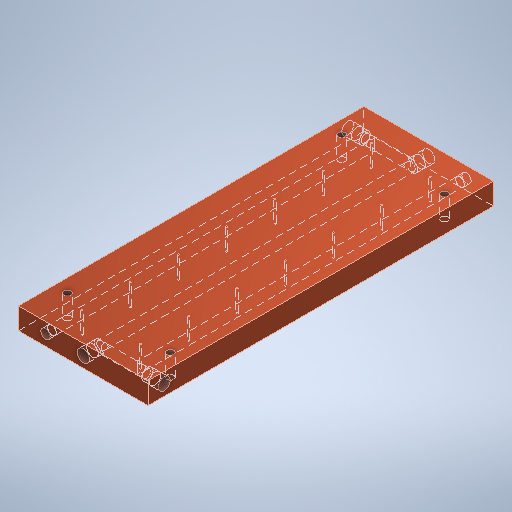
# Autodesk Inventor part: Cold Plate
Saved by Autodesk Inventor 2025 (Build 290162000, 162)
## iProperties
Created: 2025-06-10
Part Number: Cold Plate
Material: Copper
Document SubType Name: Modeling
Designer: Caleb Fangmeier
Density: 8.94 g/cm^3
Appearance: Copper - Satin
Author: Caleb Fangmeier
Autodesk Inventor part; units mm, degrees
ref_plane "YZ Plane" through (0, 0, 0) normal (1, 0, 0) x (0, 1, 0)
ref_plane "XZ Plane" through (0, 0, 0) normal (0, 1, 0) x (-1, 0, 0)
ref_plane "XY Plane" through (0, 0, 0) normal (0, 0, 1) x (1, 0, 0)
sketch "Sketch1" plane through (0, 0, 0) normal (0, 1, 0) x (-1, 0, 0)
  line L0 (-60, -160) -> (60, -160)
  line L1 (60, -160) -> (60, 160)
  line L2 (60, 160) -> (-60, 160)
  line L3 (-60, 160) -> (-60, -160)
  line L4 (-60, -160) -> (60, 160) construction
  line L5 (60, -160) -> (-60, 160) construction
  point P0 (0, 0)
  dimension "d0" = 120
  dimension "d1" = 320
  constraints: 12 end point, 2 midpoint, 2 parallel, 1 horizontal, 1 perpendicular
  measures "d0" distance of L2.end L1.end
  measures "d1" distance of L0.end L1.end
extrude "Extrusion1" add sketch "Sketch1" along normal blind 20
sketch "Right Center Hole and Plug" plane through (-60, 0, 160) normal (0, 0, 1) x (1, 0, 0)
  line L0 (120, 0) -> (120, 20) projected
  line L1 (0, 0) -> (120, 0) projected
  point P0 (60, 0)
  point P1 (60, 10)
  dimension "d4" = 60
  dimension "d5" = 10
  measures "d4" distance from line of L0 point (60, 10)
  measures "d5" distance from line of L1 point (60, 10)
hole "Hole1" at (0, 10, 160) direction (0, 0, -1) diameter 8 end through all
sketch "Back Hole and Plug" plane through (60, 0, 160) normal (1, 0, 0) x (0, 0, -1)
  line L0 (0, 0) -> (320, 0) projected
  line L1 (0, 0) -> (0, 20) projected
  point P0 (160, 0)
  point P1 (15, 10)
  dimension "d13" = 10
  dimension "d14" = 15
  measures "d13" distance from line of L0 point (15, 10)
  measures "d14" distance from line of L1 point (15, 10)
hole "Hole2" at (60, 10, 145) direction (-1, 0, 0) diameter 10.7188 depth 15.664 tip angle 118 taper from width 11.3585 to width 10.8207 over 8.6081 thread size "1/4" designation "1/4 - 18 NPT" standard "NPT for PVC Pipe and Fitting"
sketch "Front Hole and Plug" plane through (-60, 0, -160) normal (-1, 0, 0) x (0, 0, 1)
  line L0 (0, 0) -> (320, 0) projected
  line L1 (0, 0) -> (0, 20) projected
  point P0 (160, 0)
  point P1 (15, 10)
  dimension "d22" = 10
  dimension "d23" = 15
  measures "d22" distance from line of L0 point (15, 10)
  measures "d23" distance from line of point (15, 10) L1
hole "Hole3" at (-60, 10, -145) direction (1, 0, 0) diameter 10.7188 depth 15.664 tip angle 118 taper from width 11.3585 to width 10.8207 over 8.6081 thread size "1/4" designation "1/4 - 18 NPT" standard "NPT for PVC Pipe and Fitting"
sketch "Left Inlet and threading" plane through (60, 0, -160) normal (0, 0, -1) x (-1, 0, 0)
  line L0 (0, 0) -> (120, 0) projected
  line L1 (0, 0) -> (0, 20) projected
  point P0 (60, 0)
  point P1 (25, 10)
  dimension "d31" = 10
  dimension "d32" = 25
  measures "d31" distance from line of point (25, 10) L0
  measures "d32" distance from line of L1 point (25, 10)
hole "Left Inlet" at (35, 10, -160) direction (0, 0, 1) diameter 8 depth 305 tip angle 118
sketch "Right Inlet and threading" plane through (-60, 0, 160) normal (0, 0, 1) x (1, 0, 0)
  line L0 (0, 0) -> (120, 0) projected
  line L1 (0, 0) -> (0, 20) projected
  point P0 (60, 0)
  point P1 (25, 10)
  dimension "d40" = 10
  dimension "d41" = 25
  measures "d40" distance from line of L0 point (25, 10)
  measures "d41" distance from line of L1 point (25, 10)
hole "Right Inlet" at (-35, 10, 160) direction (0, 0, -1) diameter 8 depth 305 tip angle 118
hole "Hole6" at (-60, 10, -145) direction (1, 0, 0) diameter 8 depth 60 tip angle 118
hole "Hole7" at (60, 10, 145) direction (-1, 0, 0) diameter 8 depth 60 tip angle 118
hole "Hole8" at (0, 10, 160) direction (0, 0, -1) diameter 10.7188 depth 15.664 tip angle 118 taper from width 11.3585 to width 10.8207 over 8.6081 thread size "1/4" designation "1/4 - 18 NPT" standard "NPT for PVC Pipe and Fitting"
sketch "Left Center Hole and Plug" plane through (60, 0, -160) normal (0, 0, -1) x (-1, 0, 0)
  point P0 (60, 0)
  point P1 (60, 10)
hole "Hole9" at (0, 10, -160) direction (0, 0, 1) diameter 10.7188 depth 15.664 tip angle 118 taper from width 11.3585 to width 10.8207 over 8.608 thread size "1/4" designation "1/4 - 18 NPT" standard "NPT for PVC Pipe and Fitting"
hole "Hole10" at (35, 10, -160) direction (0, 0, 1) diameter 7.9502 depth 10.688 tip angle 118 taper from width 8.7371 to width 8.3632 over 5.9842 thread size "1/8" designation "1/8 - 27 NPT" standard "NPT for PVC Pipe and Fitting"
hole "Hole11" at (-35, 10, 160) direction (0, 0, -1) diameter 7.9502 depth 10.688 tip angle 118 taper from width 8.7371 to width 8.3632 over 5.984 thread size "1/8" designation "1/8 - 27 NPT" standard "NPT for PVC Pipe and Fitting"
sketch "Sketch8" plane through (0, 20, 0) normal (0, 1, 0) x (1, 0, 0)
  line L0 (60, 160) -> (-60, 160) projected
  line L1 (-60, 160) -> (-60, -160) projected
  line L2 (60, -160) -> (60, 160) projected
  line L3 (-60, -160) -> (60, -160) projected
  point P0 (0, 0)
  point P1 (-47.6, 127)
  point P2 (47.6, -127)
  point P3 (-47.6, -127)
  point P4 (47.6, 127)
  dimension "d103" = 33
  dimension "d104" = 12.4
  dimension "d105" = 12.4
  dimension "d106" = 33
  dimension "d132" = 254
  dimension "d133" = 95.2
  constraints: 2 horizontal alignment, 2 vertical alignment
  measures "d103" distance from line of L0 point (-47.6, 127)
  measures "d104" distance from line of L1 point (-47.6, 127)
  measures "d105" distance from line of L2 point (47.6, -127)
  measures "d106" distance from line of L3 point (47.6, -127)
  measures "d132" vertical distance of point (-47.6, 127) point (47.6, -127)
  measures "d133" horizontal distance of point (-47.6, 127) point (47.6, -127)
hole "Hole12" at (-47.6, 20, -127) at (47.6, 20, 127) at (-47.6, 20, 127) at (47.6, 20, -127) direction (0, -1, 0) diameter 6.647 end through all thread size "M8x1.25" class "6H" standard "ANSI Metric M Profile"
sketch "Sketch9" plane through (0, 20, 0) normal (0, 1, 0) x (1, 0, 0)
  line L0 (60, 160) -> (-60, 160) projected
  line L1 (60, -160) -> (60, 160) projected
  line L2 (-60, 160) -> (-60, -160) projected
  point P0 (0, 0)
  point P1 (27.15, 134.1)
  point P2 (27.15, 89.4)
  point P3 (27.15, 44.7)
  point P4 (27.15, 0)
  point P5 (27.15, -44.7)
  point P6 (27.15, -89.4)
  point P7 (27.15, -134.1)
  point P8 (-27.15, 134.1)
  point P9 (-27.15, 89.4)
  point P10 (-27.15, 44.7)
  point P11 (-27.15, 0)
  point P12 (-27.15, -44.7)
  point P13 (-27.15, -89.4)
  point P14 (-27.15, -134.1)
  dimension "d114" = 25.9
  dimension "d117" = 44.7
  dimension "d120" = 54.3
  dimension "d123" = 120
  dimension "d124" = 32.85
  constraints: 1 horizontal, 1 vertical, 13 other
  measures "d114" distance from line of L0 point (27.15, 134.1)
  measures "d117" distance of point (27.15, 134.1) point (27.15, 89.4)
  measures "d120" distance of point (27.15, 134.1) point (-27.15, 134.1)
  measures "d123" distance between parallel lines of L2 L1
  measures "d124" distance from line of L1 point (27.15, 134.1)
hole "Hole13" at (27.15, 20, -134.1) at (27.15, 20, -89.4) at (27.15, 20, -44.7) at (27.15, 20, 0) at (27.15, 20, 44.7) at (27.15, 20, 89.4) at (27.15, 20, 134.1) at (-27.15, 20, -134.1) at (-27.15, 20, -89.4) at (-27.15, 20, -44.7) at (-27.15, 20, 0) at (-27.15, 20, 44.7) at (-27.15, 20, 89.4) at (-27.15, 20, 134.1) direction (0, -1, 0) diameter 1.567 end through all thread size "M2x0.4" class "6H" standard "ANSI Metric M Profile"
equation "\"d105\" = d104"
equation "\"d106\" = d103"
equation "\"d124\" = -0.5 * d120 + 0.5 * d123"
body "Solid1"
